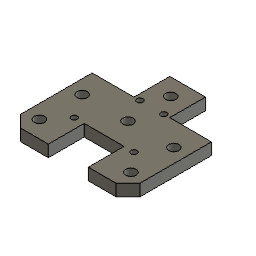
zweite_bp_ed (Autodesk Fusion 360 design; units mm, degrees)
Autodesk Fusion 360 part; units mm, degrees
note: some values were not read from the file. Set by a fixed rule: which sketch regions a step uses.
sketch "Sketch1" plane through (0, 0, 0) normal (0, 1, 0) x (1, 0, 0)
  line L0 (30, 30) -> (30, -30)
  line L1 (30, -30) -> (-30, -30)
  line L2 (-30, -30) -> (-30, 30)
  line L3 (-30, 30) -> (30, -30) construction
  line L4 (30, 30) -> (-30, -30) construction
  line L5 (10, 30) -> (10, 50)
  line L6 (10, 50) -> (-10, 50)
  line L7 (-10, 50) -> (-10, 30)
  line L8 (-30, 30) -> (-10, 30)
  line L9 (10, 30) -> (30, 30)
  circle A0 centre (0, 43) radius 2.6
  line L10 (-30, 0) -> (30, 0) construction
  circle A1 centre (0, 21.5) radius 2.6
  circle A2 centre (-23, 21.5) radius 2.6
  circle A3 centre (23, 21.5) radius 2.6
  circle A4 centre (-23, 0) radius 2.6
  circle A5 centre (0, 0) radius 2.6
  circle A6 centre (23, 0) radius 2.6
  circle A7 centre (-23, -21.5) radius 2.6
  circle A8 centre (23, -21.5) radius 2.6
  line L11 (-2.6, -21) -> (-2.6, -22)
  arc A9 (-2.6, -22) -> (2.6, -22) centre (0, -22) ccw
  line L12 (2.6, -22) -> (2.6, -21)
  arc A10 (2.6, -21) -> (-2.6, -21) centre (0, -21) ccw
  point P0 (0, -21.5)
  dimension "d4" = 60
  dimension "d5" = 60
  dimension "d7" = 20
  dimension "d8" = 20
  dimension "d9" = 5.2
  dimension "d10" = 7
  dimension "d11" = 5.2
  dimension "d12" = 21.5
  dimension "d13" = 5.2
  dimension "d14" = 5.2
  dimension "d15" = 23
  dimension "d16" = 23
  dimension "d28" = 5.2
  dimension "d29" = 0.5
  constraint horizontal L8
  constraint perpendicular L0 L9
  constraint parallel L1 L8
  constraint parallel L0 L2
  constraint coincident L3 A5.centre
  constraint coincident L4 A5.centre
  constraint coincident A5.centre origin
  constraint vertical L5
  constraint horizontal L6
  constraint vertical L7
  constraint collinear L8 L9
  constraint midpoint L2 L10.start
  constraint midpoint L0 L10.end
  constraint tangent L11 A9
  constraint tangent A9 L12
  constraint parallel L11 L12
  constraint tangent L12 A10
  constraint tangent L11 A10
  measures "d4" distance of L0.end L1.end
  measures "d5" distance of L0.start L0.end
  measures "d7" distance of L7.end L5.start
  measures "d8" distance of L7.end L6.end
  measures "d9" diameter of A0
  measures "d10" distance of L6 A0.centre
  measures "d11" diameter of A1
  measures "d12" distance of A0.centre A1.centre
  measures "d13" diameter of A2
  measures "d14" diameter of A3
  measures "d15" distance of A1.centre A2.centre
  measures "d16" distance of A1.centre A3.centre
  measures "d28" diameter of A9
  measures "d29" distance of A10.centre P0
extrude "Extrude1" add sketch "Sketch1" along normal blind 6
chamfer "Chamfer1" distance 6 angle 45 4 edges at (30, 3, 30) (30, 3, -30) (-30, 3, 30) (-30, 3, -30)
fillet "Fillet1" radius 3 2 edges at (10, 3, -50) (-10, 3, -50)
fillet "Fillet2" radius 3 2 edges at (10, 3, -30) (-10, 3, -30)
sketch "Sketch2" plane through (0, 6, 0) normal (0, 1, 0) x (-1, 0, 0)
  arc A0 (7, -50) -> (10, -47) centre (7, -47) ccw
  line L0 (10, -47) -> (10, -33)
  arc A1 (13, -30) -> (10, -33) centre (13, -33) ccw
  line L1 (13, -30) -> (24, -30)
  line L2 (24, -30) -> (30, -24)
  line L3 (30, -24) -> (30, 24)
  line L4 (30, 24) -> (24, 30)
  line L5 (24, 30) -> (-24, 30)
  line L6 (-24, 30) -> (-30, 24)
  line L7 (-30, 24) -> (-30, -24)
  line L8 (-30, -24) -> (-24, -30)
  line L9 (-24, -30) -> (-13, -30)
  arc A2 (-10, -33) -> (-13, -30) centre (-13, -33) ccw
  line L10 (-10, -33) -> (-10, -47)
  arc A3 (-10, -47) -> (-7, -50) centre (-7, -47) ccw
  line L11 (-7, -50) -> (7, -50)
  circle A4 centre (23, 0) radius 2.6
  circle A5 centre (0, 0) radius 2.6
  circle A6 centre (0, -21.5) radius 2.6
  circle A7 centre (0, -43) radius 2.6
  circle A8 centre (23, 21.5) radius 2.6
  arc A9 (-2.6, 21) -> (2.6, 21) centre (0, 21) ccw
  line L12 (-2.6, 21) -> (-2.6, 22)
  arc A10 (2.6, 22) -> (-2.6, 22) centre (0, 22) ccw
  line L13 (2.6, 22) -> (2.6, 21)
  circle A11 centre (23, -21.5) radius 2.6
  circle A12 centre (-23, 0) radius 2.6
  circle A13 centre (-23, -21.5) radius 2.6
  circle A14 centre (-23, 21.5) radius 2.6
  line L14 (10, 12) -> (-10, 12)
  line L15 (-10, 12) -> (-10, 30)
  line L16 (10, 30) -> (10, 12)
  line L17 (0, -30) -> (-9, -30)
  line L18 (0, -30) -> (9, -30)
  line L19 (9, -30) -> (9, -12)
  line L20 (-9, -30) -> (-9, -12)
  line L21 (30, -12) -> (9, -12)
  line L22 (-9, -12) -> (-30, -12)
  dimension "d40" = 20
  dimension "d41" = 18
  dimension "d44" = 10
  dimension "d45" = 9
  dimension "d46" = 9.5
  dimension "d47" = 9
  dimension "d48" = 9
  dimension "d49" = 8.5
  constraint horizontal L14
  constraint vertical L15
  constraint vertical L16
  constraint coincident L3 L21.start
  constraint coincident L7 L22.end
  constraint perpendicular L7 L22
  constraint horizontal L17
  constraint perpendicular L0 L18
  constraint perpendicular L19 L21
  constraint perpendicular L20 L22
  constraint collinear L21 L22
  measures "d40" distance of L14.start L14.end
  measures "d41" distance of L14.start L16.start
  measures "d44" distance of A10.centre L16
  measures "d45" distance of A9.centre L14
  measures "d46" distance of A6.centre L21
  measures "d47" distance of L17.start L17.end
  measures "d48" distance of L17.start L18.end
  measures "d49" distance of A6.centre L17.start
extrude "Extrude2" cut sketch "Sketch2" against normal blind 6 contours A0 L0 A1 L1 L2 L3 L7 L8 L9 A2 L10 A3 L11 L17 L18 L19 L20 L21 L22 | L5 L14 L15 L16
sketch "Sketch3" plane through (0, 6, 0) normal (0, 1, 0) x (-1, 0, 0)
  circle A0 centre (0, 0) radius 2.6
  circle A1 centre (23, 21.5) radius 2.6
  circle A2 centre (0, -21.5) radius 2.6
  circle A3 centre (23, 0) radius 2.6
  circle A4 centre (-23, 0) radius 2.6
  circle A5 centre (-23, 21.5) radius 2.6
  line L0 (10, 30) -> (10, 12)
  line L1 (10, 12) -> (-10, 12)
  line L2 (-10, 12) -> (-10, 30)
  line L3 (-10, 30) -> (-24, 30)
  line L4 (-24, 30) -> (-30, 24)
  line L5 (-30, 24) -> (-30, -12)
  line L6 (-30, -12) -> (-9, -12)
  line L7 (-9, -12) -> (-9, -30)
  line L8 (-9, -30) -> (9, -30)
  line L9 (9, -30) -> (9, -12)
  line L10 (9, -12) -> (30, -12)
  line L11 (30, -12) -> (30, 24)
  line L12 (30, 24) -> (24, 30)
  line L13 (24, 30) -> (10, 30)
  circle A6 centre (15, 12) radius 1.5
  circle A7 centre (-15, 12) radius 1.5
  circle A8 centre (6, -11.9995) radius 1.5
  circle A9 centre (-6, -11.9995) radius 1.5
  dimension "d53" = 3
  dimension "d54" = 15
  dimension "d55" = 12
  dimension "d56" = 3
  dimension "d57" = 15
  dimension "d58" = 12
  dimension "d59" = 3
  dimension "d60" = 3
  dimension "d61" = 6
  dimension "d62" = 6
  dimension "d63" = 13.416
  dimension "d64" = 13.416
  measures "d53" diameter of A6
  measures "d54" horizontal distance of A0.centre A6.centre
  measures "d55" vertical distance of A0.centre A6.centre
  measures "d56" diameter of A7
  measures "d57" horizontal distance of A0.centre A7.centre
  measures "d58" vertical distance of A0.centre A7.centre
  measures "d59" diameter of A8
  measures "d60" diameter of A9
  measures "d61" horizontal distance of A0.centre A9.centre
  measures "d62" horizontal distance of A0.centre A8.centre
  measures "d63" distance of A0.centre A8.centre
  measures "d64" distance of A0.centre A9.centre
extrude "Extrude3" cut sketch "Sketch3" against normal blind 6 contours A6 | A7 | A8 | A9
equation "larger_hole_radii = 2.6 mm"
equation "small_hole_Radii = 1.25 mm"
equation "base_sqaure_dim = 60 mm"
equation "d4 = base_sqaure_dim"
equation "d5 = base_sqaure_dim"
equation "square_extension = 20 mm"
equation "d7 = square_extension"
equation "d8 = square_extension"
equation "d9 = larger_hole_radii * 2"
equation "d11 = larger_hole_radii * 2"
equation "d13 = 2 * larger_hole_radii"
equation "d14 = 2 * larger_hole_radii"
equation "dist_between_Rows = 21.50 mm"
equation "slot_height = 5.20 mm"
equation "slot_width = 0.50 mm"
equation "d28 = slot_height"
equation "d29 = slot_width"
equation "ext = 6.0 mm"
equation "d31 = ext"
equation "d33 = ext"
equation "fillet_top = 3 mm"
equation "d36 = fillet_top"
equation "d38 = fillet_top"
equation "slot_square_cutout_height = 18 mm"
equation "d40 = square_extension"
equation "d41 = slot_square_cutout_height"
equation "d44 = square_extension / 2"
equation "d45 = slot_square_cutout_height / 2"
equation "d46 = square_extension / 2 - 0.50 mm"
equation "d47 = slot_square_cutout_height / 2"
equation "d48 = slot_square_cutout_height / 2"
equation "d49 = slot_square_cutout_height / 2 - 0.50 mm"
equation "d50 = -ext"
equation "new_small_hole_dia = 3 mm"
equation "d53 = new_small_hole_dia"
equation "d56 = new_small_hole_dia"
equation "d59 = new_small_hole_dia"
equation "d60 = new_small_hole_dia"
equation "d65 = -ext"
